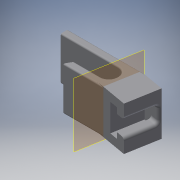
# Autodesk Inventor part: pinza0.4
Saved by Autodesk Inventor 2016 (Build 200138000, 138)
## iProperties
Created: 2015-12-16
Part Number: pinza0.4
Material: Generic
Document SubType Name: Modeling
Designer: pc
Density: 1 g/cm^3
Appearance: Default
Author: pc
Autodesk Inventor part; units mm, degrees
ref_plane "YZ Plane" through (0, 0, 0) normal (1, 0, 0) x (0, 1, 0)
ref_plane "XZ Plane" through (0, 0, 0) normal (0, 1, 0) x (-1, 0, 0)
ref_plane "XY Plane" through (0, 0, 0) normal (0, 0, 1) x (1, 0, 0)
sketch "Sketch1" plane through (0, 0, 0) normal (0, 0, 1) x (1, 0, 0)
  line L0 (-14.2044, 2.5) -> (-2.5, 2.5)
  line L1 (-2.5, 2.5) -> (-2.5, 8.5)
  line L2 (-2.5, 8.5) -> (-14.2044, 8.5)
  line L3 (-25, 11) -> (0, 11)
  line L4 (0, 11) -> (0, 0)
  line L5 (0, 0) -> (-15.6271, 0)
  line L6 (-14.2044, 2.5) -> (-15.6271, 0)
  line L7 (-14.2044, 8.5) -> (-25, 8.5)
  line L8 (-25, 8.5) -> (-25, 11)
  dimension "d4" = 6
  dimension "d22" = 25
  dimension "d23" = 11
  dimension "d24" = 11.7044
  dimension "d27" = 15.6271
  dimension "d28" = 11.7044
  dimension "d29" = 2.5
  dimension "d30" = 2.5
  constraints: 18 end point, 3 perpendicular, 2 horizontal, 1 coincident, 1 other
  measures "d4" distance of L0.end L1.end
  measures "d22" distance of L3.start L3.end
  measures "d23" distance of L3.end L4.end
  measures "d24" distance of L1.end L2.end
  measures "d27" distance of L5.end point (0, 0)
  measures "d28" distance of L0.start L0.end
  measures "d29" distance of L7.end L3.start
  measures "d30" distance from line of L4 L0.end
extrude "Extrusion1" add sketch "Sketch1" along normal blind 15
ref_plane "Work Plane1" through (0, 11, 0) normal (0.9848078, -0.1736482, 0) x (0, 0, 1)
sketch "Sketch3" plane through (0, 0, 0) normal (0, 0, -1) x (-1, 0, 0)
  line L0 (3.1619, -6.9323) -> (-0.527, 13.9887) projected
  line L1 (2.5, 2.5) -> (14.2044, 2.5) projected
  line L2 (2.5, 8.5) -> (2.5, 2.5) projected
  line L3 (25, 8.5) -> (2.5, 8.5) projected
  line L4 (0, 11) -> (25, 11) projected
  line L5 (0, 0) -> (0, 11) projected
  line L6 (15.6271, 0) -> (0, 0) projected
  line L7 (25, 0) -> (0, 0) projected
  line L8 (1.9396, 0) -> (0, 0)
  line L9 (0, 0) -> (0, 11)
  line L10 (0, 11) -> (1.9396, 0)
  line L11 (25, 11) -> (25, 8.5) projected
  line L12 (14.2044, 2.5) -> (15.6271, 0) projected
  constraints: 6 end point, 2 point on line, 1 collinear, 1 perpendicular
extrude "Extrusion2" cut sketch "Sketch3" against normal blind 20 contours L6 L5 L0
sketch "Sketch4" plane through (-1.4988, 2.5, 15) normal (0.9848078, -0.1736482, 0) x (0, 0, 1)
  line L0 (0, 2.5386) -> (0, -8.6311) projected
  line L1 (-15, 2.5386) -> (0, 2.5386) projected
  line L2 (-15, -8.6311) -> (-15, 2.5386) projected
  line L3 (-15, -8.6311) -> (-15, 2.5386) projected
  line L4 (-15, -8.6311) -> (0, -8.6311) projected
  line L5 (0, 2.5386) -> (0, -8.6311) projected
  line L6 (-15, 2.5386) -> (-15, -8.6311)
  line L7 (-15, -8.6311) -> (0, -8.6311)
  line L8 (0, -8.6311) -> (0, 2.5386)
  line L9 (-15, 2.5386) -> (0, 2.5386) projected
  line L10 (-15, -8.6311) -> (0, -8.6311) projected
  point P0 (-15, 2.2018)
  constraints: 6 end point, 1 collinear, 1 perpendicular, 1 vertical
extrude "Extrusion3" add sketch "Sketch4" along normal blind 1
sketch "Sketch6" plane through (-1.9396, 0, 0) normal (-0.1736482, -0.9848078, 0) x (0.9848078, -0.1736482, 0)
  line L0 (1, 15) -> (1, 0) projected
  line L1 (1, 15) -> (8.8, 15)
  line L2 (8.8, 15) -> (8.8, 10.2)
  line L3 (8.8, 10.2) -> (5.8, 10.2)
  line L4 (5.8, 10.2) -> (5.8, 12.2)
  line L5 (5.8, 12.2) -> (3, 12.2)
  line L6 (3, 12.2) -> (3, 2.8)
  line L7 (3, 2.8) -> (5.8, 2.8)
  line L8 (5.8, 2.8) -> (5.8, 4.8)
  line L9 (5.8, 4.8) -> (8.8, 4.8)
  line L10 (8.8, 4.8) -> (8.8, 0)
  line L11 (8.8, 0) -> (1, 0)
  line L12 (1, 0) -> (1, 15)
  point P0 (1.9101, 0)
  dimension "d13" = 5.4
  dimension "d14" = 2
  dimension "d15" = 2
  dimension "d16" = 2.8
  dimension "d17" = 3
  constraints: 24 end point, 9 perpendicular, 4 point on line, 2 collinear, 1 horizontal
  measures "d13" distance of L9.end L2.end
  measures "d14" distance of L3.end L4.end
  measures "d15" distance between parallel lines of L0 L6
  measures "d16" distance of L6.end L7.end
  measures "d17" distance of L8.end L9.end
extrude "Extrusion4" add sketch "Sketch6" against normal up to surface (11.1697 mm away)
sketch "Sketch7" plane through (0, 11, 15) normal (0.1736482, 0.9848078, 0) x (0.9848078, -0.1736482, 0)
  line L0 (0, 15) -> (0, 0) projected
  line L1 (0, 0) -> (8.8, 0) projected
  line L2 (8.8, 4.8) -> (8.8, 0) projected
  line L3 (5.8, 4.8) -> (8.8, 4.8) projected
  line L4 (5.8, 2.8) -> (5.8, 4.8) projected
  line L5 (3, 2.8) -> (5.8, 2.8) projected
  line L6 (3, 12.2) -> (3, 2.8) projected
  line L7 (5.8, 12.2) -> (3, 12.2) projected
  line L8 (5.8, 10.2) -> (5.8, 12.2) projected
  line L9 (8.8, 10.2) -> (5.8, 10.2) projected
  line L10 (8.8, 15) -> (8.8, 10.2) projected
  line L11 (0, 15) -> (8.8, 15) projected
  line L12 (8.8, 4.8) -> (8.8, 0) projected
  line L13 (3, 12.2) -> (8.8, 12.2)
  line L14 (8.8, 12.2) -> (8.8, 2.6)
  line L15 (8.8, 2.6) -> (3, 2.6)
  line L16 (3, 2.6) -> (3, 12.2)
  point P0 (1.9101, 15)
  constraints: 8 end point, 2 parallel, 1 horizontal, 1 perpendicular, 1 point on line
extrude "Extrusion5" add sketch "Sketch7" against normal blind 1 contours L10 L9 L8 L13 | L15 L16 L5 L4 L3 L2 | L14 L3 L4 L5 L6 L7 L8 L9
fillet "Fillet3" radius 1 5 edges at (7.6097, 3.4795, 4.8) (7.6097, 3.4795, 10.2) (7.0154, 8.7476, 10.2) (7.0154, 8.7476, 4.8) (8.4927, 8.4871, 7.5)
fillet "Fillet1" radius 2.8 2 edges at (-2.5, 2.5, 7.5) (-2.5, 8.5, 7.5)
fillet "Fillet2" radius 0.5 17 edges at (-9.7522, 2.5, 0) (-9.7522, 2.5, 15) (-9.7522, 8.5, 15) (-19.6022, 8.5, 15) (-9.7522, 8.5, 0) (-19.6022, 8.5, 0) (-25, 11, 7.5) (-12.5, 11, 0) (-12.5, 11, 15) (-8.7833, 0, 0) (-8.7833, 0, 15) (-3.3201, 3.3201, 0) (-3.3201, 3.3201, 15) (-2.5, 5.5, 0) (-2.5, 5.5, 15) (-3.3201, 7.6799, 0) (-3.3201, 7.6799, 15)
body "Solid1"
